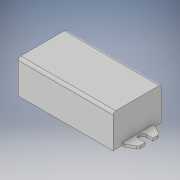
# Autodesk Inventor part: Drok-DC-9v+-to-5v-Converter
Saved by Autodesk Inventor 2017 (Build 210142000, 142)
## iProperties
Created: 2018-04-08
Part Number: Drok-DC-9v+-to-5v-Converter
Material: Generic
Document SubType Name: Modeling
Designer: MtgSaber
Density: 1 g/cm^3
Appearance: Default
Author: MtgSaber
Autodesk Inventor part; units mm, degrees
ref_plane "YZ Plane" through (0, 0, 0) normal (1, 0, 0) x (0, 1, 0)
ref_plane "XZ Plane" through (0, 0, 0) normal (0, 1, 0) x (-1, 0, 0)
ref_plane "XY Plane" through (0, 0, 0) normal (0, 0, 1) x (1, 0, 0)
sketch "Sketch1" plane through (0, 0, 0) normal (0, 1, 0) x (-1, 0, 0)
  line L0 (29.3688, 15.0812) -> (-29.3688, 15.0812)
  line L1 (-29.3688, 15.0812) -> (-29.3688, -15.0812)
  line L2 (-29.3688, -15.0812) -> (29.3688, -15.0812)
  line L3 (29.3688, -15.0812) -> (29.3688, 15.0812)
  line L4 (41.1163, 0) -> (-41.1162, 0) construction
  line L5 (0, -21.1137) -> (0, 21.1137) construction
  point P0 (0, 0)
  point P1 (0, -15.0812)
  point P2 (29.3688, 0)
  dimension "d0" = 58.7375
  dimension "d1" = 30.1625
  constraints: 8 end point, 2 midpoint, 2 parallel, 2 point on line, 1 horizontal, 1 perpendicular
  measures "d0" distance of L1.end L2.end
  measures "d1" distance of L0.end L1.end
extrude "Extrusion1" add sketch "Sketch1" along normal blind 20.6375
sketch "Sketch3" plane through (0, 0, 0) normal (0, 1, 0) x (-1, 0, 0)
  line L0 (-29.3688, 15.0812) -> (-29.3688, -15.0812) construction
  line L1 (41.1163, 0) -> (-41.1163, 0) construction
  line L2 (-29.3688, 9.525) -> (-29.3688, -9.525)
  line L3 (-29.3688, -9.525) -> (-30.9563, -9.525)
  line L4 (-30.9563, -9.525) -> (-35.7126, -6.8071)
  arc A0 (-32.5438, -2.3813) -> (-32.5438, 2.3813) centre (-32.5438, 0) ccw
  line L5 (-32.5438, -2.3813) -> (-36.5125, -2.3813)
  line L6 (-36.5125, -5.4287) -> (-36.5125, -2.3813)
  line L7 (-29.3688, 9.525) -> (-30.9563, 9.525)
  line L8 (-30.9563, 9.525) -> (-35.7126, 6.8071)
  line L9 (-32.5438, 2.3813) -> (-36.5125, 2.3813)
  line L10 (-36.5125, 5.4287) -> (-36.5125, 2.3813)
  arc A1 (-36.5125, -5.4287) -> (-35.7126, -6.8071) centre (-34.925, -5.4287) ccw
  arc A2 (-35.7126, 6.8071) -> (-36.5125, 5.4287) centre (-34.925, 5.4287) ccw
  point P0 (0, 0)
  point P1 (-29.3688, 0)
  point P2 (-36.5125, -6.35)
  point P3 (-30.1625, 0)
  point P4 (-36.5125, 6.35)
  dimension "d4" = 19.05
  dimension "d5" = 1.5875
  dimension "d6" = 7.1437
  dimension "d7" = 6.35
  dimension "d9" = 4.7625
  dimension "d10" = 6.35
  dimension "d11" = 1.5875
  dimension "d12" = 1.5875
  constraints: 18 end point, 7 point on circle, 7 point on line, 5 tangent, 4 symmetric about line, 3 centre point, 2 vertical, 1 collinear, 1 horizontal, 1 midpoint, 1 perpendicular
  measures "d4" distance of L2.start L2.end
  measures "d5" distance of L2.end L3.end
  measures "d6" distance from line of L2 point (-36.513, -6.35)
  measures "d7" distance from line of L1 point (-36.513, -6.35)
  measures "d9" diameter of A0
  measures "d10" horizontal distance of L5.end point (-30.163, 0)
  measures "d11" radius of A1
  measures "d12" radius of A2
extrude "Extrusion2" add sketch "Sketch3" along normal blind 1.5875
mirror "Mirror1" about plane through (0, 0, 0) normal (1, 0, 0) of "Extrusion2"
fillet "Fillet1" radius 1.5875 2 edges at (0, 20.6375, 15.0812) (0, 20.6375, -15.0812)
body "Solid1"
